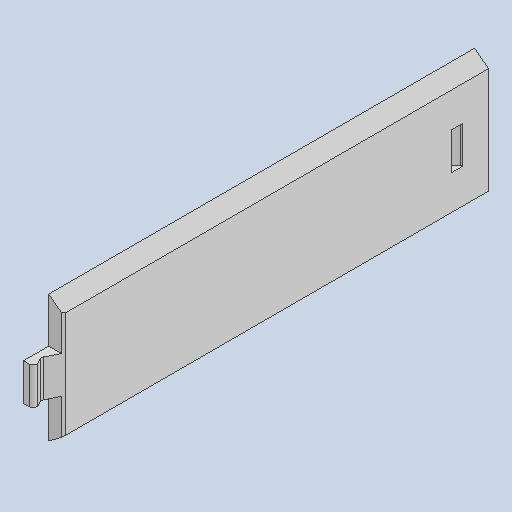
# Autodesk Inventor part: enclosure cover
Saved by Autodesk Inventor 2022 (Build 260153000, 153)
## iProperties
Created: 2021-10-08
Part Number: enclosure cover
Material: Generic
Document SubType Name: Modeling
Designer: tecware
Density: 1 g/cm^3
Appearance: Default
Author: tecware
## iProperties of the stored document enclosure cover_3DPrint.ipt
Created: 2021-10-11
Part Number: enclosure cover_3DPrint
Material: Generic
Document SubType Name: Modeling
Designer: tecware
Density: 1 g/cm^3
Appearance: Default
Author: tecware
Autodesk Inventor part; units mm, degrees
ref_plane "YZ Plane" through (0, 0, 0) normal (1, 0, 0) x (0, 1, 0)
ref_plane "XZ Plane" through (0, 0, 0) normal (0, 1, 0) x (-1, 0, 0)
ref_plane "XY Plane" through (0, 0, 0) normal (0, 0, 1) x (1, 0, 0)
ref_plane "Work Plane3" through (0, -2, -2) normal (0, 0, -1) x (-1, 0, 0)
sketch "Sketch4" plane through (0, -2, -2) normal (0, 0, -1) x (-1, 0, 0)
  line L0 (-30, 33) -> (-30, 34) projected
  line L1 (3, -2) -> (-26, -2) projected
  line L2 (7, 2) -> (7, 34) projected
  line L3 (3, 38) -> (-26, 38) projected
  line L4 (-27, 17.5) -> (-42, 17.5)
  line L5 (-30, 3.2) -> (-26, 0.2)
  line L6 (-26.2, 0.2) -> (-26.2, 17.5)
  line L7 (-30, 3.2) -> (-30, 17.5)
  line L8 (-30, 31.8) -> (-26, 34.8)
  line L9 (-26.2, 34.8) -> (-26.2, 17.5)
  line L10 (-30, 31.8) -> (-30, 17.5)
  line L11 (-26.2, 3.2) -> (-25.2, 3.2)
  line L12 (-25.2, 3.2) -> (-25.2, 17.5)
  line L13 (-26.2, 31.8) -> (-25.2, 31.8)
  line L14 (-25.2, 31.8) -> (-25.2, 17.5)
  circle A0 centre (-11.5, 18) radius 8 projected
  arc A1 (3, -2) -> (7, 2) centre (3, 2) ccw projected
  arc A2 (7, 34) -> (3, 38) centre (3, 34) ccw projected
  arc A3 (-26, 38) -> (-30, 34) centre (-26, 34) ccw projected
  line L15 (-30, 33) -> (-26, 36) projected
  line L16 (-26, 36) -> (-26, 0) projected
  line L17 (-26, 0) -> (-30, 3) projected
  line L18 (-30, 2) -> (-30, 3) projected
  arc A4 (-30, 2) -> (-26, -2) centre (-26, 2) ccw projected
  point P0 (0, 2)
  point P1 (-26.2, 0.35)
  point P2 (-26.2, 34.65)
  point P3 (-26.2, 31.8)
  point P4 (-26, 33)
  point P5 (-26, 2)
  dimension "d55" = 1
  dimension "d56" = 4
  dimension "d57" = 3
  dimension "d59" = 3.8
  constraints: 22 end point, 5 symmetric about line, 3 point on line, 2 horizontal, 1 perpendicular
  measures "d55" distance of L11.start L11.end
  measures "d56" horizontal distance of L5.start L5.end
  measures "d57" vertical distance of L5.start L5.end
  measures "d59" distance between parallel lines of L7 L6
extrude "Whole Cover" add sketch "Sketch4" against normal blind 122 contours L9 L6 L5 L7 L10 L8
ref_plane "Work Plane4" through (0, 15.5, 120) normal (0, -1, 0) x (0, 0, -1)
sketch "Sketch5" plane through (0, 15.5, 120) normal (0, -1, 0) x (0, 0, -1)
  line L0 (122, 30) -> (0, 30) projected
  line L1 (122, 26.2) -> (0, 26.2) projected
  line L2 (0, 26.2) -> (0, 30)
  line L3 (7.85, 30) -> (-0.75, 30)
  line L4 (3.55, 30) -> (3.55, 27.8)
  line L5 (3.0945, 28.033) -> (-0.75, 30)
  line L6 (4.0055, 28.033) -> (7.85, 30)
  arc A0 (3.0945, 28.033) -> (4.0055, 28.033) centre (3.55, 28.9233) ccw
  point P0 (120, 0)
  point P1 (0, 29.6163)
  point P2 (0, 30)
  dimension "d45" = 8.6
  dimension "d47" = 2.2
  dimension "d48" = 1
  constraints: 10 end point, 3 point on line, 2 point on circle, 2 tangent, 1 centre point, 1 collinear, 1 midpoint, 1 vertical
  measures "d45" distance of L3.start L3.end
  measures "d47" distance of L4.start L4.end
  measures "d48" radius of A0
extrude "Snap fit" cut sketch "Sketch5" along normal through all both and the other way through all
sketch "Sketch6" plane through (30, 1.2, -2) normal (1, 0, 0) x (0, 0, -1)
  line L0 (0, -2.85) -> (0, 31.45) projected
  line L1 (0, 14.3) -> (-7, 14.3) construction
  line L2 (-7, 9.3) -> (-10, 9.3)
  line L3 (-10, 9.3) -> (-10, 19.3)
  line L4 (-10, 19.3) -> (-7, 19.3)
  line L5 (-7, 19.3) -> (-7, 9.3)
  point P0 (-2, -1.2)
  dimension "d15" = 3
  dimension "d16" = 10
  dimension "d17" = 7
  constraints: 10 end point, 2 horizontal, 2 midpoint, 2 parallel, 2 perpendicular
  measures "d15" distance of L3.end L4.end
  measures "d16" distance of L2.end L3.end
  measures "d17" distance between parallel lines of L0 L5
extrude "Grip" cut sketch "Sketch6" against normal blind 2
chamfer "Grip Chamfer" distance 1.5 angle 45 2 edges at (28, 15.5, 8) (28, 15.5, 5)
sketch "Sketch9" plane through (30, 1.2, -2) normal (1, 0, 0) x (0, 0, -1)
  line L0 (0, 0) -> (-122, 0) projected
  line L1 (-122, 31.45) -> (-122, -2.85) projected
  line L2 (-122, 14.3) -> (-114.6731, 14.3)
  line L3 (0, -2.85) -> (-122, -2.85) projected
  line L4 (-122, -2.85) -> (-114.5, -2.85)
  line L5 (-114.5, -2.85) -> (-114.5, 0.15)
  line L6 (-114.5, 0.15) -> (-122, 0.15)
  line L7 (-122, 0.15) -> (-122, -2.85)
  line L8 (-122, 31.45) -> (-114.5, 31.45)
  line L9 (-114.5, 31.45) -> (-114.5, 28.45)
  line L10 (-114.5, 28.45) -> (-122, 28.45)
  line L11 (-122, 28.45) -> (-122, 31.45)
  line L12 (-122, 28.45) -> (-121.6, 28.45)
  line L13 (-121.6, 28.45) -> (-121.6, 0.15)
  line L14 (-121.6, 0.15) -> (-122, 0.15)
  line L15 (-122, 0.15) -> (-122, 28.45)
  line L16 (-117.25, 0.15) -> (-117.25, -2.85)
  line L17 (-117.25, 28.45) -> (-117.25, 31.45)
  line L18 (-114.5, 9.3) -> (-122.5, 9.3)
  line L19 (-122.5, 9.3) -> (-122.5, 19.3)
  line L20 (-122.5, 19.3) -> (-114.5, 19.3)
  line L21 (-114.5, 19.3) -> (-114.5, 9.3)
  line L22 (-114.5, 0.15) -> (-114.5, 9.3)
  line L23 (-114.5, 19.3) -> (-114.5, 28.45)
  line L24 (-114.8, -2.85) -> (-114.8, 9.3)
  line L25 (-114.8, 31.45) -> (-114.8, 19.3)
  point P0 (-2, -1.2)
  point P1 (-117.25, 0)
  point P2 (-117.25, 28.6)
  point P3 (-122, 28.6)
  point P4 (-117.25, 0)
  point P5 (-114.5, 0)
  point P6 (-121.6, 9.3)
  point P7 (-121.6, 19.3)
  point P8 (-114.8, 19.3)
  dimension "d41" = 7.5
  dimension "d42" = 3
  dimension "d43" = 0.4
  dimension "d44" = 2.75
  dimension "d49" = 8
  dimension "d50" = 10
  dimension "d60" = 0.3
  constraints: 46 end point, 8 symmetric about line, 6 parallel, 5 perpendicular, 5 point on line, 4 horizontal, 2 collinear, 1 midpoint
  measures "d41" distance of L6.end L5.end
  measures "d42" distance of L5.end L4.end
  measures "d43" distance of L13.end L14.end
  measures "d44" distance between parallel lines of L5 L16
  measures "d49" distance of L19.end L20.end
  measures "d50" distance of L18.end L19.end
  measures "d60" distance between parallel lines of L22 L24
extrude "Corner Cut" cut sketch "Sketch9" against normal through all contours L24 L3 L16 L0 | L0 L16 L6 L24 | L16 L3 L1 L0 | L0 L1 L6 L16 | L6 L13 L18 L24 | L1 L18 L13 L6 | L18 L1 L2 L13 | L20 L13 L10 L25 | L2 L1 L20 L13 | L20 L1 L10 L13 | L10 L17 L8 L25 | L10 L1 L8 L17
fillet "Fillet5" radius 1 1 edges at (29.4116, 15.5, 119.6)
body "Solid2"
